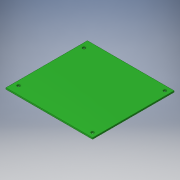
# Autodesk Inventor part: PC 104 size and hole model
Saved by Autodesk Inventor 2016 (Build 200138000, 138)
## iProperties
Created: 2016-10-03
Part Number: PC 104 size and hole model
Material: FR-4
Document SubType Name: Modeling
Designer: R.P. SMITH
Mass: 25.4983 g
Surface Area: 178.878 cm^2
Volume: 13.7828 cm^3
Density: 1.85 g/cm^3
Appearance: Smooth - Dark Forest Green
Author: R.P. SMITH
Autodesk Inventor part; units mm, degrees
ref_plane "YZ Plane" through (0, 0, 0) normal (1, 0, 0) x (0, 1, 0)
ref_plane "XZ Plane" through (0, 0, 0) normal (0, 1, 0) x (-1, 0, 0)
ref_plane "XY Plane" through (0, 0, 0) normal (0, 0, 1) x (1, 0, 0)
sketch "Sketch1" plane through (0, 0, 0) normal (0, 1, 0) x (-1, 0, 0)
  line L0 (47.9425, 45.085) -> (-47.9425, 45.085)
  line L1 (-47.9425, 45.085) -> (-47.9425, -45.085)
  line L2 (-47.9425, -45.085) -> (47.9425, -45.085)
  line L3 (47.9425, -45.085) -> (47.9425, 45.085)
  line L4 (47.9425, 45.085) -> (-47.9425, -45.085) construction
  line L5 (-47.9425, 45.085) -> (47.9425, -45.085) construction
  circle A0 centre (42.8625, 36.195) radius 1.5875
  circle A1 centre (42.8625, -36.195) radius 1.5875
  circle A2 centre (-42.8625, -40.005) radius 1.5875
  circle A3 centre (-42.8625, 40.005) radius 1.5875
  point P0 (0, 0)
  dimension "d0" = 90.17
  dimension "d1" = 95.885
  dimension "d2" = 5.08
  dimension "d3" = 5.08
  dimension "d4" = 5.08
  dimension "d5" = 8.89
  dimension "d6" = 8.89
  dimension "d7" = 5.08
  dimension "d8" = 3.175
  dimension "d9" = 3.175
  dimension "d10" = 3.175
  dimension "d11" = 3.175
  constraints: 12 end point, 4 centre point, 4 coincident, 2 midpoint, 2 parallel, 2 vertical alignment, 1 horizontal, 1 perpendicular
  measures "d0" distance of L0.end L1.end
  measures "d1" distance of L0.start L0.end
  measures "d2" distance from line of L0 point (-42.862, 40.005)
  measures "d3" distance from line of L2 point (-42.862, -40.005)
  measures "d4" distance from line of L1 point (-42.862, -40.005)
  measures "d5" distance from line of L0 point (42.863, 36.195)
  measures "d6" distance from line of L2 point (42.863, -36.195)
  measures "d7" distance from line of L3 point (42.863, -36.195)
  measures "d8" diameter of A0
  measures "d9" diameter of A1
  measures "d10" diameter of A2
  measures "d11" diameter of A3
extrude "Extrusion1" add sketch "Sketch1" along normal mid plane 1.6
equation "\"d7\" = d4"
equation "\"d9\" = d8"
equation "\"d10\" = d8"
equation "\"d11\" = d8"
body "Solid1"
